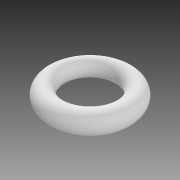
# Autodesk Inventor part: oring_5x7
Saved by Autodesk Inventor 2020 (Build 240168000, 168)
## iProperties
Created: 2020-11-28
Part Number: oring_5x7
Material: Generic
Document SubType Name: Modeling
Designer: DDeGo
Density: 1 g/cm^3
Appearance: Default
Author: DDeGo
Autodesk Inventor part; units mm, degrees
ref_plane "YZ Plane" through (0, 0, 0) normal (1, 0, 0) x (0, 1, 0)
ref_plane "XZ Plane" through (0, 0, 0) normal (0, 1, 0) x (-1, 0, 0)
ref_plane "XY Plane" through (0, 0, 0) normal (0, 0, 1) x (1, 0, 0)
sketch "Sketch1" plane through (0, 0, 0) normal (0, 0, 1) x (1, 0, 0)
  line L0 (0, 1.1669) -> (0, 0) construction
  line L1 (0, 0) -> (2.75, 0) construction
  circle A0 centre (2.75, 0) radius 0.75
  line L2 (2, 0.4543) -> (2, -0.4265) construction
  dimension "d0" = 1.5
  dimension "d1" = 2
  constraints: 6 end point, 2 vertical, 1 centre point, 1 coincident, 1 perpendicular, 1 tangent
  measures "d0" diameter of A0
  measures "d1" distance between parallel lines of L0 L2
revolve "Revolution1" add sketch "Sketch1" angle 360 about axis through (0, 1.1669, 0) along (0, -1, 0)
body "Solid1"
